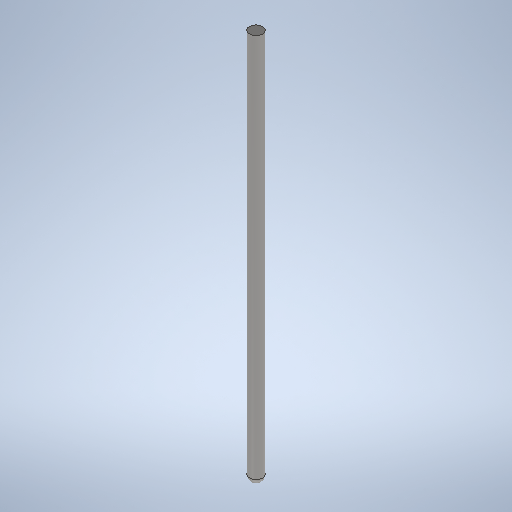
# Autodesk Inventor part: Impactorv2
Saved by Autodesk Inventor 2025 (Build 290162000, 162)
## iProperties
Created: 2025-07-14
Part Number: Impactorv2
Material: Steel, Carbon
Document SubType Name: Modeling
Designer: dr1e22
Density: 681.576 g/cm^3
Appearance: Semi-Polished
Mass: 11694 g
Surface Area: 240.772 cm^2
Volume: 94.9683 cm^3
Author: dr1e22
Autodesk Inventor part; units mm, degrees
ref_plane "YZ Plane" through (0, 0, 0) normal (1, 0, 0) x (0, 1, 0)
ref_plane "XZ Plane" through (0, 0, 0) normal (0, 1, 0) x (-1, 0, 0)
ref_plane "XY Plane" through (0, 0, 0) normal (0, 0, 1) x (1, 0, 0)
sketch "Sketch1" plane through (0, 0, 0) normal (0, 1, 0) x (-1, 0, 0)
  arc A0 (-8, 0) -> (8, 0) centre (0, 0) ccw
  line L0 (8, 0) -> (-8, 0)
  dimension "d0" = 16
  constraints: 2 end point, 2 point on circle, 1 centre point, 1 coincident, 1 horizontal
  measures "d0" diameter of A0
revolve "Revolution1" add sketch "Sketch1" angle 180 about axis through (-8, 0, 0) along (-1, 0, 0)
sketch "Sketch2" plane through (0, 0, 0) normal (0, 1, 0) x (1, 0, 0)
  point P0 (0, 0)
sketch "Sketch3" plane through (0, 0, 0) normal (0, 1, 0) x (1, 0, 0)
  circle A0 centre (0, 0) radius 8
  dimension "d2" = 16
  constraints: 1 centre point, 1 coincident
  measures "d2" diameter of A0
extrude "Extrusion1" add sketch "Sketch3" along normal blind 467
body "Solid1"
